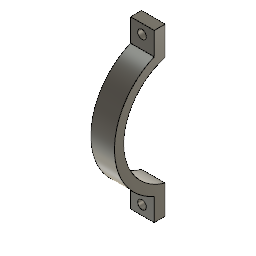
moter brackets v1 (Autodesk Fusion 360 design; units mm, degrees)
Autodesk Fusion 360 part; units mm, degrees
note: some values were not read from the file. Set by a fixed rule: which sketch regions a step uses.
sketch "Sketch3" plane through (80.4545, 0, 0) normal (1, 0, 0) x (0, 0, -1)
  arc A0 (13.2129, 0) -> (13.2129, 6.35) centre (0, 3.175) ccw
  line L0 (13.2129, 6.35) -> (-13.2129, 6.35)
  arc A1 (-13.2129, 6.35) -> (-13.2129, 0) centre (0, 3.175) ccw
  line L1 (-13.2129, 0) -> (13.2129, 0)
  circle A2 centre (0, 3.175) radius 12.0015
  circle A3 centre (0, 3.175) radius 12.0015
  circle A4 centre (0, 3.175) radius 12.0269
  dimension "d1" = 24.0538
  measures "d1" diameter of A4
sketch "Sketch4" plane through (0, 6.35, 0) normal (0, 1, 0) x (-1, 0, 0)
  line L0 (-58.42, -11.6002) -> (-75.2536, -11.6002)
  line L1 (-75.2536, -11.6002) -> (-75.2536, -13.7183)
  line L2 (-75.2536, -13.7183) -> (-80.4545, -13.7183)
  line L3 (-80.4545, -13.7183) -> (-80.4545, -13.2129)
  line L4 (-80.4545, -13.2129) -> (-103.5685, -13.2129)
  line L5 (-103.5685, -13.2129) -> (-103.5685, -15.494)
  arc A0 (-103.5685, -15.494) -> (-101.9232, -17.6884) centre (-101.2825, -15.494) ccw
  arc A1 (-100.2964, -19.5934) -> (-101.9232, -17.6884) centre (-102.564, -19.8827) ccw
  arc A2 (-100.2964, -19.5934) -> (-98.0287, -21.59) centre (-98.0287, -19.304) ccw
  line L6 (-98.0287, -21.59) -> (-97.4568, -21.59)
  arc A3 (-97.4568, -21.59) -> (-95.2028, -19.685) centre (-97.4568, -19.304) ccw
  arc A4 (-92.9487, -17.78) -> (-95.2028, -19.685) centre (-92.9487, -20.066) ccw
  line L7 (-92.9487, -17.78) -> (-89.8368, -17.78)
  arc A5 (-87.5828, -19.685) -> (-89.8368, -17.78) centre (-89.8368, -20.066) ccw
  arc A6 (-87.5828, -19.685) -> (-85.3287, -21.59) centre (-85.3287, -19.304) ccw
  line L8 (-85.3287, -21.59) -> (-84.8207, -21.59)
  arc A7 (-84.8207, -21.59) -> (-82.5667, -19.685) centre (-84.8207, -19.304) ccw
  arc A8 (-80.3127, -17.78) -> (-82.5667, -19.685) centre (-80.3127, -20.066) ccw
  line L9 (-80.3127, -17.78) -> (-51.816, -17.78)
  arc A9 (-49.53, -20.066) -> (-51.816, -17.78) centre (-51.816, -20.066) ccw
  line L10 (-49.53, -20.066) -> (-49.53, -32.004)
  arc A10 (-49.53, -32.004) -> (-47.244, -34.29) centre (-47.244, -32.004) ccw
  line L11 (-47.244, -34.29) -> (-33.9568, -34.29)
  arc A11 (-31.7028, -36.195) -> (-33.9568, -34.29) centre (-33.9568, -36.576) ccw
  arc A12 (-31.7028, -36.195) -> (-29.4487, -38.1) centre (-29.4487, -35.814) ccw
  line L12 (-29.4487, -38.1) -> (-28.9407, -38.1)
  arc A13 (-28.9407, -38.1) -> (-26.6867, -36.195) centre (-28.9407, -35.814) ccw
  arc A14 (-24.4327, -34.29) -> (-26.6867, -36.195) centre (-24.4327, -36.576) ccw
  line L13 (-24.4327, -34.29) -> (-21.2568, -34.29)
  arc A15 (-19.0028, -36.195) -> (-21.2568, -34.29) centre (-21.2568, -36.576) ccw
  arc A16 (-19.0028, -36.195) -> (-16.7487, -38.1) centre (-16.7487, -35.814) ccw
  line L14 (-16.7487, -38.1) -> (-16.1768, -38.1)
  arc A17 (-16.1768, -38.1) -> (-13.9228, -36.195) centre (-16.1768, -35.814) ccw
  arc A18 (-11.6687, -34.29) -> (-13.9228, -36.195) centre (-11.6687, -36.576) ccw
  line L15 (-11.6687, -34.29) -> (11.7327, -34.29)
  arc A19 (13.9867, -36.195) -> (11.7327, -34.29) centre (11.7327, -36.576) ccw
  arc A20 (13.9867, -36.195) -> (16.2407, -38.1) centre (16.2407, -35.814) ccw
  line L16 (16.2407, -38.1) -> (16.7487, -38.1)
  arc A21 (16.7487, -38.1) -> (19.0028, -36.195) centre (16.7487, -35.814) ccw
  arc A22 (21.2568, -34.29) -> (19.0028, -36.195) centre (21.2568, -36.576) ccw
  line L17 (21.2568, -34.29) -> (24.4327, -34.29)
  arc A23 (26.6867, -36.195) -> (24.4327, -34.29) centre (24.4327, -36.576) ccw
  arc A24 (26.6867, -36.195) -> (28.9407, -38.1) centre (28.9407, -35.814) ccw
  curve K0
  arc A25 (29.5127, -38.1) -> (31.7667, -36.195) centre (29.5127, -35.814) ccw
  arc A26 (34.0207, -34.29) -> (31.7667, -36.195) centre (34.0207, -36.576) ccw
  line L18 (34.0207, -34.29) -> (47.244, -34.29)
  arc A27 (47.244, -34.29) -> (49.53, -32.004) centre (47.244, -32.004) ccw
  line L19 (49.53, -32.004) -> (49.53, -20.066)
  arc A28 (51.816, -17.78) -> (49.53, -20.066) centre (51.816, -20.066) ccw
  line L20 (51.816, -17.78) -> (82.5347, -17.78)
  line L21 (82.5347, -17.78) -> (82.5347, -19.304)
  arc A29 (82.5347, -19.304) -> (84.8207, -21.59) centre (84.8207, -19.304) ccw
  line L22 (84.8207, -21.59) -> (85.3287, -21.59)
  arc A30 (85.3287, -21.59) -> (87.5828, -19.685) centre (85.3287, -19.304) ccw
  arc A31 (89.8368, -17.78) -> (87.5828, -19.685) centre (89.8368, -20.066) ccw
  line L23 (89.8368, -17.78) -> (93.0127, -17.78)
  arc A32 (95.2667, -19.685) -> (93.0127, -17.78) centre (93.0127, -20.066) ccw
  arc A33 (95.2667, -19.685) -> (97.5207, -21.59) centre (97.5207, -19.304) ccw
  line L24 (97.5207, -21.59) -> (98.0287, -21.59)
  arc A34 (98.0287, -21.59) -> (100.3147, -19.304) centre (98.0287, -19.304) ccw
  line L25 (100.3147, -19.304) -> (100.3147, -17.78)
  line L26 (100.3147, -17.78) -> (101.2825, -17.78)
  arc A35 (101.2825, -17.78) -> (103.5685, -15.494) centre (101.2825, -15.494) ccw
  line L27 (103.5685, -15.494) -> (103.5685, -13.2129)
  line L28 (103.5685, -13.2129) -> (80.4545, -13.2129)
  line L29 (80.4545, -13.2129) -> (80.4545, -13.7183)
  line L30 (80.4545, -13.7183) -> (75.3745, -13.7183)
  line L31 (75.3745, -13.7183) -> (75.3745, -11.6002)
  line L32 (75.3745, -11.6002) -> (58.42, -11.6002)
  line L33 (58.42, -11.6002) -> (58.42, -13.7183)
  line L34 (58.42, -13.7183) -> (53.34, -13.7183)
  line L35 (53.34, -13.7183) -> (53.34, -11.6002)
  line L36 (53.34, -11.6002) -> (47.4345, -11.6002)
  line L37 (47.4345, -11.6002) -> (47.4345, -11.5644)
  spline S0 degree 3 poles (46.3169, -10.2511) (46.3169, -10.4171) (46.3545, -10.6128) (46.4774, -10.9167) (46.583, -11.0795) (46.8063, -11.3079) (46.9623, -11.4151) (47.2052, -11.5178) (47.3211, -11.5502) (47.4345, -11.5644) knots 0.578205 0.578205 0.578205 0.578205 0.628019 0.628019 0.676542 0.676542 0.723852 0.723852 0.755663 0.755663 0.755663 0.755663
  line L38 (46.3169, -10.2511) -> (46.3169, 10.2511)
  spline S1 degree 3 poles (47.4345, 11.5644) (47.3211, 11.5502) (47.2052, 11.5178) (46.9623, 11.4151) (46.8063, 11.3079) (46.583, 11.0795) (46.4774, 10.9167) (46.3545, 10.6128) (46.3169, 10.4171) (46.3169, 10.2511) knots 0.014624 0.014624 0.014624 0.014624 0.046435 0.046435 0.093744 0.093744 0.142267 0.142267 0.192082 0.192082 0.192082 0.192082
  line L39 (47.4345, 11.5644) -> (47.4345, 11.6002)
  line L40 (47.4345, 11.6002) -> (53.34, 11.6002)
  line L41 (53.34, 11.6002) -> (53.34, 13.7183)
  line L42 (53.34, 13.7183) -> (58.42, 13.7183)
  line L43 (58.42, 13.7183) -> (58.42, 11.6002)
  line L44 (58.42, 11.6002) -> (75.3745, 11.6002)
  line L45 (75.3745, 11.6002) -> (75.3745, 13.7183)
  line L46 (75.3745, 13.7183) -> (80.4545, 13.7183)
  line L47 (80.4545, 13.7183) -> (80.4545, 13.2129)
  line L48 (80.4545, 13.2129) -> (103.5685, 13.2129)
  line L49 (103.5685, 13.2129) -> (103.5685, 15.494)
  arc A36 (103.5685, 15.494) -> (101.2825, 17.78) centre (101.2825, 15.494) ccw
  line L50 (101.2825, 17.78) -> (100.3147, 17.78)
  line L51 (100.3147, 17.78) -> (100.3147, 19.304)
  arc A37 (100.3147, 19.304) -> (98.0287, 21.59) centre (98.0287, 19.304) ccw
  line L52 (98.0287, 21.59) -> (97.4568, 21.59)
  arc A38 (97.4568, 21.59) -> (95.2028, 19.685) centre (97.4568, 19.304) ccw
  arc A39 (92.9487, 17.78) -> (95.2028, 19.685) centre (92.9487, 20.066) ccw
  line L53 (92.9487, 17.78) -> (89.9007, 17.78)
  arc A40 (87.6467, 19.685) -> (89.9007, 17.78) centre (89.9007, 20.066) ccw
  arc A41 (87.6467, 19.685) -> (85.3927, 21.59) centre (85.3927, 19.304) ccw
  line L54 (85.3927, 21.59) -> (84.7568, 21.59)
  arc A42 (84.7568, 21.59) -> (82.5028, 19.685) centre (84.7568, 19.304) ccw
  arc A43 (80.2487, 17.78) -> (82.5028, 19.685) centre (80.2487, 20.066) ccw
  line L55 (80.2487, 17.78) -> (51.816, 17.78)
  arc A44 (49.53, 20.066) -> (51.816, 17.78) centre (51.816, 20.066) ccw
  line L56 (49.53, 20.066) -> (49.53, 32.004)
  arc A45 (49.53, 32.004) -> (47.244, 34.29) centre (47.244, 32.004) ccw
  line L57 (47.244, 34.29) -> (33.9568, 34.29)
  arc A46 (31.7028, 36.195) -> (33.9568, 34.29) centre (33.9568, 36.576) ccw
  arc A47 (31.7028, 36.195) -> (29.4487, 38.1) centre (29.4487, 35.814) ccw
  curve K1
  arc A48 (28.8768, 38.1) -> (26.6228, 36.195) centre (28.8768, 35.814) ccw
  arc A49 (24.3687, 34.29) -> (26.6228, 36.195) centre (24.3687, 36.576) ccw
  line L58 (24.3687, 34.29) -> (21.2568, 34.29)
  arc A50 (19.0028, 36.195) -> (21.2568, 34.29) centre (21.2568, 36.576) ccw
  arc A51 (19.0028, 36.195) -> (16.7487, 38.1) centre (16.7487, 35.814) ccw
  line L59 (16.7487, 38.1) -> (16.1768, 38.1)
  arc A52 (16.1768, 38.1) -> (13.9228, 36.195) centre (16.1768, 35.814) ccw
  arc A53 (11.6687, 34.29) -> (13.9228, 36.195) centre (11.6687, 36.576) ccw
  line L60 (11.6687, 34.29) -> (-11.7327, 34.29)
  arc A54 (-13.9867, 36.195) -> (-11.7327, 34.29) centre (-11.7327, 36.576) ccw
  arc A55 (-13.9867, 36.195) -> (-16.2407, 38.1) centre (-16.2407, 35.814) ccw
  line L61 (-16.2407, 38.1) -> (-16.8127, 38.1)
  arc A56 (-16.8127, 38.1) -> (-19.0667, 36.195) centre (-16.8127, 35.814) ccw
  arc A57 (-21.3207, 34.29) -> (-19.0667, 36.195) centre (-21.3207, 36.576) ccw
  line L62 (-21.3207, 34.29) -> (-24.4327, 34.29)
  arc A58 (-26.6867, 36.195) -> (-24.4327, 34.29) centre (-24.4327, 36.576) ccw
  arc A59 (-26.6867, 36.195) -> (-28.9407, 38.1) centre (-28.9407, 35.814) ccw
  curve K2
  arc A60 (-29.5127, 38.1) -> (-31.7667, 36.195) centre (-29.5127, 35.814) ccw
  arc A61 (-34.0207, 34.29) -> (-31.7667, 36.195) centre (-34.0207, 36.576) ccw
  line L63 (-34.0207, 34.29) -> (-47.244, 34.29)
  arc A62 (-47.244, 34.29) -> (-49.53, 32.004) centre (-47.244, 32.004) ccw
  line L64 (-49.53, 32.004) -> (-49.53, 20.066)
  arc A63 (-51.816, 17.78) -> (-49.53, 20.066) centre (-51.816, 20.066) ccw
  line L65 (-51.816, 17.78) -> (-82.5347, 17.78)
  line L66 (-82.5347, 17.78) -> (-82.5347, 19.304)
  arc A64 (-82.5347, 19.304) -> (-84.8207, 21.59) centre (-84.8207, 19.304) ccw
  line L67 (-84.8207, 21.59) -> (-85.3927, 21.59)
  arc A65 (-85.3927, 21.59) -> (-87.6467, 19.685) centre (-85.3927, 19.304) ccw
  arc A66 (-89.9007, 17.78) -> (-87.6467, 19.685) centre (-89.9007, 20.066) ccw
  line L68 (-89.9007, 17.78) -> (-95.2347, 17.78)
  line L69 (-95.2347, 17.78) -> (-95.2347, 19.304)
  arc A67 (-95.2347, 19.304) -> (-97.5207, 21.59) centre (-97.5207, 19.304) ccw
  line L70 (-97.5207, 21.59) -> (-98.0287, 21.59)
  arc A68 (-98.0287, 21.59) -> (-100.2828, 19.685) centre (-98.0287, 19.304) ccw
  arc A69 (-101.9097, 17.8677) -> (-100.2828, 19.685) centre (-102.5368, 20.066) ccw
  arc A70 (-101.9097, 17.8677) -> (-103.5685, 15.6694) centre (-101.2825, 15.6694) ccw
  line L71 (-103.5685, 15.6694) -> (-103.5685, 13.2129)
  line L72 (-103.5685, 13.2129) -> (-80.4545, 13.2129)
  line L73 (-80.4545, 13.2129) -> (-80.4545, 13.7183)
  line L74 (-80.4545, 13.7183) -> (-75.2536, 13.7183)
  line L75 (-75.2536, 13.7183) -> (-75.2536, 11.6002)
  line L76 (-75.2536, 11.6002) -> (-58.42, 11.6002)
  line L77 (-58.42, 11.6002) -> (-58.42, 13.7183)
  line L78 (-58.42, 13.7183) -> (-53.34, 13.7183)
  line L79 (-53.34, 13.7183) -> (-53.34, 11.6002)
  line L80 (-53.34, 11.6002) -> (-47.4345, 11.6002)
  line L81 (-47.4345, 11.6002) -> (-47.4345, 11.5644)
  spline S2 degree 3 poles (-46.3169, 10.2511) (-46.3169, 10.4171) (-46.3545, 10.6128) (-46.4774, 10.9167) (-46.583, 11.0795) (-46.8063, 11.3079) (-46.9623, 11.4151) (-47.2052, 11.5178) (-47.3211, 11.5502) (-47.4345, 11.5644) knots 0.578205 0.578205 0.578205 0.578205 0.628019 0.628019 0.676542 0.676542 0.723852 0.723852 0.755663 0.755663 0.755663 0.755663
  line L82 (-46.3169, 10.2511) -> (-46.3169, -10.2511)
  spline S3 degree 3 poles (-47.4345, -11.5644) (-47.3211, -11.5502) (-47.2052, -11.5178) (-46.9623, -11.4151) (-46.8063, -11.3079) (-46.583, -11.0795) (-46.4774, -10.9167) (-46.3545, -10.6128) (-46.3169, -10.4171) (-46.3169, -10.2511) knots 0.014624 0.014624 0.014624 0.014624 0.046435 0.046435 0.093744 0.093744 0.142267 0.142267 0.192082 0.192082 0.192082 0.192082
  line L83 (-47.4345, -11.5644) -> (-47.4345, -11.6002)
  line L84 (-47.4345, -11.6002) -> (-53.34, -11.6002)
  line L85 (-53.34, -11.6002) -> (-53.34, -13.7183)
  line L86 (-53.34, -13.7183) -> (-58.42, -13.7183)
  line L87 (-58.42, -13.7183) -> (-58.42, -11.6002)
  line L88 (99.06, 17.78) -> (96.52, 17.78)
  line L89 (96.52, 17.78) -> (96.52, 20.32)
  line L90 (96.52, 20.32) -> (99.06, 20.32)
  line L91 (99.06, 20.32) -> (99.06, 17.78)
  line L92 (86.36, 17.78) -> (83.82, 17.78)
  line L93 (83.82, 17.78) -> (83.82, 20.32)
  line L94 (83.82, 20.32) -> (86.36, 20.32)
  line L95 (86.36, 20.32) -> (86.36, 17.78)
  line L96 (-86.36, -17.78) -> (-83.82, -17.78)
  line L97 (-83.82, -17.78) -> (-83.82, -20.32)
  line L98 (-83.82, -20.32) -> (-86.36, -20.32)
  line L99 (-86.36, -20.32) -> (-86.36, -17.78)
  line L100 (-99.06, -17.78) -> (-96.52, -17.78)
  line L101 (-96.52, -17.78) -> (-96.52, -20.32)
  line L102 (-96.52, -20.32) -> (-99.06, -20.32)
  line L103 (-99.06, -20.32) -> (-99.06, -17.78)
  line L104 (-30.48, -34.29) -> (-27.94, -34.29)
  line L105 (-27.94, -34.29) -> (-27.94, -36.83)
  line L106 (-27.94, -36.83) -> (-30.48, -36.83)
  line L107 (-30.48, -36.83) -> (-30.48, -34.29)
  line L108 (-15.24, -34.29) -> (-15.24, -36.83)
  line L109 (-15.24, -36.83) -> (-17.78, -36.83)
  line L110 (-17.78, -36.83) -> (-17.78, -34.29)
  line L111 (-17.78, -34.29) -> (-15.24, -34.29)
  line L112 (17.78, -34.29) -> (17.78, -36.83)
  line L113 (17.78, -36.83) -> (15.24, -36.83)
  line L114 (15.24, -36.83) -> (15.24, -34.29)
  line L115 (15.24, -34.29) -> (17.78, -34.29)
  line L116 (30.48, -34.29) -> (30.48, -36.83)
  line L117 (30.48, -36.83) -> (27.94, -36.83)
  line L118 (27.94, -36.83) -> (27.94, -34.29)
  line L119 (27.94, -34.29) -> (30.48, -34.29)
  line L120 (-30.48, 34.29) -> (-30.48, 36.83)
  line L121 (-30.48, 36.83) -> (-27.94, 36.83)
  line L122 (-27.94, 36.83) -> (-27.94, 34.29)
  line L123 (-27.94, 34.29) -> (-30.48, 34.29)
  line L124 (30.48, 34.29) -> (27.94, 34.29)
  line L125 (27.94, 34.29) -> (27.94, 36.83)
  line L126 (27.94, 36.83) -> (30.48, 36.83)
  line L127 (30.48, 36.83) -> (30.48, 34.29)
  line L128 (-17.78, 34.29) -> (-17.78, 36.83)
  line L129 (-17.78, 36.83) -> (-15.24, 36.83)
  line L130 (-15.24, 36.83) -> (-15.24, 34.29)
  line L131 (-15.24, 34.29) -> (-17.78, 34.29)
  line L132 (17.78, 34.29) -> (15.24, 34.29)
  line L133 (15.24, 34.29) -> (15.24, 36.83)
  line L134 (15.24, 36.83) -> (17.78, 36.83)
  line L135 (17.78, 36.83) -> (17.78, 34.29)
  line L136 (-99.06, 17.78) -> (-99.06, 20.32)
  line L137 (-99.06, 20.32) -> (-96.52, 20.32)
  line L138 (-96.52, 20.32) -> (-96.52, 17.78)
  line L139 (-96.52, 17.78) -> (-99.06, 17.78)
  line L140 (-86.36, 17.78) -> (-86.36, 20.32)
  line L141 (-86.36, 20.32) -> (-83.82, 20.32)
  line L142 (-83.82, 20.32) -> (-83.82, 17.78)
  line L143 (-83.82, 17.78) -> (-86.36, 17.78)
  line L144 (86.36, -17.78) -> (86.36, -20.32)
  line L145 (86.36, -20.32) -> (83.82, -20.32)
  line L146 (83.82, -20.32) -> (83.82, -17.78)
  line L147 (83.82, -17.78) -> (86.36, -17.78)
  line L148 (99.06, -17.78) -> (99.06, -20.32)
  line L149 (99.06, -20.32) -> (96.52, -20.32)
  line L150 (96.52, -20.32) -> (96.52, -17.78)
  line L151 (96.52, -17.78) -> (99.06, -17.78)
  line L152 (-80.4545, 13.7183) -> (-75.2536, 13.7183)
  line L153 (-75.2536, 13.7183) -> (-75.2536, 17.78)
  line L154 (-75.2536, 17.78) -> (-80.4545, 17.78)
  line L155 (-80.4545, 17.78) -> (-80.4545, 13.7183)
  line L156 (-58.42, 13.7183) -> (-53.34, 13.7183)
  line L157 (-53.34, 13.7183) -> (-53.34, 17.78)
  line L158 (-53.34, 17.78) -> (-58.42, 17.78)
  line L159 (-58.42, 17.78) -> (-58.42, 13.7183)
  line L160 (-58.42, -13.7183) -> (-53.34, -13.7183)
  line L161 (-53.34, -13.7183) -> (-53.34, -17.78)
  line L162 (-53.34, -17.78) -> (-58.42, -17.78)
  line L163 (-58.42, -17.78) -> (-58.42, -13.7183)
  line L164 (-80.4545, -13.7183) -> (-75.2536, -13.7183)
  line L165 (-75.2536, -13.7183) -> (-75.2536, -17.78)
  line L166 (-75.2536, -17.78) -> (-80.4545, -17.78)
  line L167 (-80.4545, -17.78) -> (-80.4545, -13.7183)
  line L168 (0.032, -34.29) -> (-0.032, 34.29) construction
  circle A71 centre (-55.88, -15.7491) radius 0.8001
  line L169 (-55.88, 15.7492) -> (-55.88, -15.7491)
  line L170 (-80.4545, 13.7183) -> (-75.2536, 13.7183)
  line L171 (-75.2536, 13.7183) -> (-75.2536, 17.78)
  line L172 (-75.2536, 17.78) -> (-80.4545, 17.78)
  line L173 (-80.4545, 17.78) -> (-80.4545, 13.7183)
  line L174 (-77.854, 15.7492) -> (-55.88, 15.7492)
  circle A72 centre (-77.851, -15.7491) radius 0.8001
  circle A73 centre (-55.88, 15.7469) radius 0.8001
  circle A74 centre (-77.851, 15.7469) radius 0.8001
  circle A75 centre (77.8215, 15.892) radius 0.8001
  circle A76 centre (55.8505, 15.851) radius 0.8001
  circle A77 centre (55.9093, -15.6449) radius 0.8001
  circle A78 centre (77.8802, -15.6039) radius 0.8001
  dimension "d2" = 1.6002
  dimension "d3" = 21.974
  dimension "d4" = 31.4983
  measures "d2" diameter of A71
sketch "Sketch1" plane through (80.4545, -4.4132, 0) normal (1, 0, 0) x (0, 0, -1)
  arc A0 (-11.6002, 4.4132) -> (11.6002, 4.4133) centre (0, 7.6228) ccw
  circle A1 centre (0, 7.5882) radius 12.0015
  circle A2 centre (0, 7.5882) radius 12.0015
  arc A3 (13.7183, 10.7632) -> (-13.7183, 10.7632) centre (0, 7.5882) ccw
  arc A4 (13.7183, 10.7632) -> (-13.7183, 10.7633) centre (0, 7.5882) ccw
  arc A5 (-12.9062, 2.0427) -> (12.9062, 2.0427) centre (0, 7.6228) ccw
  line L0 (-17.78, 4.4196) -> (-17.7837, 2.0502)
  line L1 (-17.7837, 2.0502) -> (-12.9062, 2.0427)
  line L2 (0, 4.4132) -> (0, -6.438) construction
  line L3 (17.78, 4.4196) -> (17.7837, 2.0502)
  line L4 (17.7837, 2.0502) -> (12.9062, 2.0427)
  line L5 (-11.6002, 4.4132) -> (-17.78, 4.4196)
  line L6 (11.6002, 4.4132) -> (17.78, 4.4196)
  dimension "d122" = 0
  dimension "d123" = 0
  dimension "d124" = 0
  dimension "d125" = 0
  dimension "d134" = 0
  dimension "d135" = 0
  dimension "d136" = 0
  dimension "d137" = 0
  dimension "d146" = 0
  dimension "d147" = 0
  dimension "d148" = 0
  dimension "d149" = 0
  dimension "d158" = 0
  dimension "d159" = 0
  dimension "d160" = 0
  dimension "d161" = 0
extrude "Extrude1" add sketch "Sketch1" against normal blind 5.08 contours A0 A5 L0 L1 L3 L4 L5 L6
move_face "MoveFace1" to x (1, 0, 0) y (0, 1, 0) z (0, 0, 1) at (-24.13, 0, 0) 1 faces at (77.0678, -2.989, -12.6208)
extrude "Extrude2" cut sketch "Sketch4" against normal blind 6.35 contours L169 L174 A73 | L169 L174 A73 | A71 | A72 | A74 | A75 | A76 | A77 | A78
sketch "Sketch2" plane through (0, -2.3905, 0.0037) normal (0, -0.999999, 0.001542) x (1, 0, 0)
  line L0 (80.4545, 12.9025) -> (80.4545, 17.78)
  line L1 (80.4545, 17.78) -> (75.3745, 17.78)
  line L2 (75.3745, 17.78) -> (75.3745, 12.9025)
  line L3 (75.3745, 12.9025) -> (80.4545, 12.9025)
  ellipse E0 centre (77.851, 15.7468) end of major axis (77.0509, 15.7468) minor radius 0.8001
  circle A0 centre (77.851, 15.7468) radius 0.9271
  line L4 (80.4545, -17.7873) -> (80.4545, -12.9098)
  line L5 (80.4545, -12.9098) -> (75.3745, -12.9098)
  line L6 (75.3745, -12.9098) -> (75.3745, -17.7873)
  line L7 (75.3745, -17.7873) -> (80.4545, -17.7873)
  ellipse E1 centre (77.851, -15.7491) end of major axis (77.0509, -15.7491) minor radius 0.8001
  circle A1 centre (77.851, -15.7491) radius 0.9271
  dimension "d72" = 1.8542
  dimension "d73" = 1.8542
  measures "d72" diameter of A0
  measures "d73" diameter of A1
extrude "Extrude3" cut sketch "Sketch2" against normal blind 2.54 contours E0 | A0 | E1 | A1
